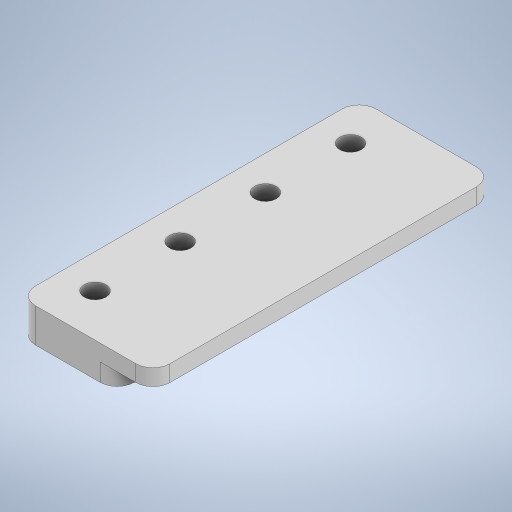
# Autodesk Inventor part: FMR_DXWD80_CPW_Halter_D
Saved by Autodesk Inventor 2023 (Build 270158000, 158)
## iProperties
Created: 2023-05-16
Part Number: FMR_DXWD80_CPW_Halter_D
Material: Generisch
Document SubType Name: Modeling
Designer: Markus Meinert
Density: 1 g/cm^3
Appearance: Vorgabe
Author: Markus Meinert
Autodesk Inventor part; units mm, degrees
ref_plane "YZ Plane" through (0, 0, 0) normal (1, 0, 0) x (0, 1, 0)
ref_plane "XZ Plane" through (0, 0, 0) normal (0, 1, 0) x (-1, 0, 0)
ref_plane "XY Plane" through (0, 0, 0) normal (0, 0, 1) x (1, 0, 0)
sketch "Skizze1" plane through (0, 0, 0) normal (0, 0, 1) x (1, 0, 0)
  line L0 (-10.2503, 0) -> (-10.2503, 10)
  line L1 (-10.2503, 10) -> (29.2497, 10)
  line L2 (29.2497, 10) -> (29.2497, 5.2)
  line L3 (29.2497, 5.2) -> (18.7497, 5.2)
  line L4 (18.7497, 5.2) -> (18.7497, 0)
  line L5 (18.7497, 0) -> (-10.2503, 0)
  point P0 (0, 0)
  dimension "d0" = 39.5
  dimension "d1" = 10
  dimension "d2" = 5.2
  dimension "d5" = 10.5
  constraints: 12 end point, 5 perpendicular, 1 vertical
  measures "d0" distance of L0.end L1.end
  measures "d1" distance of L0.start L0.end
  measures "d2" distance of L3.end L4.end
  measures "d5" distance of L2.end L3.end
extrude "Extrusion1" add sketch "Skizze1" along normal blind 100
sketch "Skizze2" plane through (-10.2503, 10, 0) normal (0, 1, 0) x (1, 0, 0)
  line L0 (0, 0) -> (0, -100) projected
  line L1 (39.5, 0) -> (39.5, -100) projected
  line L2 (39.5, -100) -> (0, -100) projected
  point P0 (10.2503, 0)
  point P1 (10, -37.5)
  point P2 (10, -62.5)
  point P3 (10, -87.5)
  point P4 (10, -12.5)
  dimension "d10" = 10
  dimension "d11" = 10
  dimension "d12" = 10
  dimension "d13" = 12.5
  dimension "d14" = 25
  dimension "d15" = 25
  dimension "d16" = 10
  dimension "d17" = 25
  measures "d10" distance from line of L0 point (10, -37.5)
  measures "d11" distance from line of L0 point (10, -62.5)
  measures "d12" distance from line of L0 point (10, -87.5)
  measures "d13" distance from line of L2 point (10, -87.5)
  measures "d14" distance of point (10, -62.5) point (10, -87.5)
  measures "d15" distance of point (10, -37.5) point (10, -62.5)
  measures "d16" distance from line of L0 point (10, -12.5)
  measures "d17" distance of point (10, -37.5) point (10, -12.5)
hole "Bohrung1" at (-0.2503, 10, 37.5) at (-0.2503, 10, 62.5) at (-0.2503, 10, 87.5) at (-0.2503, 10, 12.5) direction (0, -1, 0) diameter 6.4 end through all
fillet "Rundung1" radius 5 6 edges at (-10.2503, 5, 0) (-10.2503, 5, 100) (29.2497, 7.6, 0) (18.7497, 2.6, 0) (29.2497, 7.6, 100) (18.7497, 2.6, 100)
